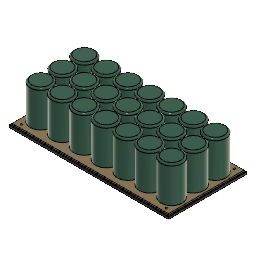
Condensadores (Autodesk Fusion 360 design; units mm, degrees)
Autodesk Fusion 360 part; units mm, degrees
sketch "Esboço1" plane through (0, 0, 0) normal (0, 0, 1) x (1, 0, 0)
  line L0 (0, 0) -> (230, 0)
  line L1 (230, 0) -> (230, 113)
  line L2 (230, 113) -> (0, 113)
  line L3 (0, 113) -> (0, 0)
  dimension "d1" = 230
  dimension "d2" = 113
  constraint horizontal L0
  constraint vertical L1
  constraint horizontal L2
  constraint vertical L3
  constraint coincident L0.start L3.end
  measures "d1" distance of L1.end L2.end
  measures "d2" distance of L0.start L2.end
extrude "Extrusão1" add sketch "Esboço1" along normal blind 3.5 makes body 1
sketch "Esboço2" plane through (0, 0, 3.5) normal (0, 0, 1) x (-1, 0, 0)
  line L0 (0, -113) -> (0, 0)
  line L1 (0, 0) -> (-230, 0)
  line L2 (-230, 0) -> (-230, -113)
  line L3 (-230, -113) -> (0, -113)
  line L4 (-2, -111) -> (-228, -111)
  line L5 (-228, -111) -> (-228, -2)
  line L6 (-228, -2) -> (-2, -2)
  line L7 (-2, -2) -> (-2, -111)
  line L8 (0, -113) -> (0, 0)
  line L9 (-230, -113) -> (0, -113)
  line L10 (-230, 0) -> (-230, -113)
  line L11 (0, 0) -> (-230, 0)
  circle A0 centre (-10.5, -105.5) radius 1.5
  circle A1 centre (-219.5, -105.5) radius 1.5
  circle A2 centre (-10.5, -7.5) radius 1.5
  circle A3 centre (-219.5, -7.5) radius 1.5
  circle A4 centre (-209.5, -88) radius 15.25
  circle A5 centre (-209.5, -56.5) radius 15.25
  circle A6 centre (-209.5, -25) radius 15.25
  line L12 (-209.5, -88) -> (-209.5, -56.5) construction
  line L13 (-209.5, -56.5) -> (-209.5, -25) construction
  line L14 (-209.5, -88) -> (-2, -88) construction
  line L15 (-209.5, -25) -> (-2, -25) construction
  line L16 (-209.5, -56.5) -> (-2, -56.5) construction
  circle A7 centre (-20.5, -88) radius 15.25
  circle A8 centre (-20.5, -56.5) radius 15.25
  circle A9 centre (-20.5, -25) radius 15.25
  circle A10 centre (-52, -25) radius 15.25
  circle A11 centre (-83.5, -25) radius 15.25
  circle A12 centre (-146.5, -25) radius 15.25
  circle A13 centre (-178, -25) radius 15.25
  circle A14 centre (-178, -56.5) radius 15.25
  circle A15 centre (-115, -56.5) radius 15.25
  circle A16 centre (-146.5, -56.5) radius 15.25
  circle A17 centre (-83.5, -56.5) radius 15.25
  circle A18 centre (-52, -56.5) radius 15.25
  circle A19 centre (-52, -88) radius 15.25
  circle A20 centre (-83.5, -88) radius 15.25
  circle A21 centre (-115, -88) radius 15.25
  circle A22 centre (-146.5, -88) radius 15.25
  circle A23 centre (-178, -88) radius 15.25
  circle A24 centre (-115, -25) radius 15.25
  line L17 (-178, -88) -> (-178, -2) construction
  line L18 (-146.5, -88) -> (-146.5, -2) construction
  line L19 (-115, -88) -> (-115, -2) construction
  line L20 (-83.5, -88) -> (-83.5, -2) construction
  line L21 (-52, -88) -> (-52, -2) construction
  line L22 (-20.5, -88) -> (-20.5, -2) construction
  dimension "d5" = 2
  dimension "d6" = 2
  dimension "d7" = 2
  dimension "d8" = 2
  dimension "d9" = 3
  dimension "d10" = 3
  dimension "d11" = 3
  dimension "d12" = 3
  dimension "d13" = 10.5
  dimension "d14" = 7.5
  dimension "d15" = 10.5
  dimension "d16" = 7.5
  dimension "d17" = 7.5
  dimension "d18" = 10.5
  dimension "d19" = 10.5
  dimension "d20" = 7.5
  dimension "d21" = 30.5
  dimension "d22" = 18.5
  dimension "d23" = 23
  dimension "d24" = 23
  dimension "d25" = 31.5
  dimension "d26" = 31.5
  dimension "d27" = 31.5
  dimension "d28" = 31.5
  dimension "d29" = 31.5
  dimension "d30" = 31.5
  dimension "d31" = 31.5
  dimension "d32" = 31.5
  constraint horizontal L4
  constraint vertical L5
  constraint horizontal L6
  constraint vertical L7
  constraint equal A4 A6
  constraint equal A4 A5
  constraint coincident A4.centre L12.start
  constraint coincident A5.centre L12.end
  constraint coincident A6.centre L13.end
  constraint vertical L12
  constraint vertical L13
  constraint coincident L7 L14.end
  constraint perpendicular L7 L14
  constraint coincident L7 L15.end
  constraint perpendicular L7 L15
  constraint coincident L7 L16.end
  constraint coincident L14 A7.centre
  constraint coincident L16 A8.centre
  constraint coincident L15 A9.centre
  constraint coincident L15 A10.centre
  constraint coincident L15 A11.centre
  constraint coincident L15 A13.centre
  constraint coincident L16 A14.centre
  constraint coincident L16 A18.centre
  constraint coincident L14 A19.centre
  constraint coincident L14 A20.centre
  constraint coincident L14 A21.centre
  constraint coincident L14 A22.centre
  constraint coincident L14 A23.centre
  constraint equal A22 A23
  constraint equal A21 A22
  constraint equal A20 A21
  constraint equal A19 A20
  constraint equal A7 A19
  constraint equal A4 A7
  constraint coincident L16 A15.centre
  constraint equal A8 A18
  constraint equal A8 A17
  constraint equal A15 A17
  constraint equal A15 A16
  constraint equal A14 A16
  constraint equal A5 A14
  constraint coincident L15 A12.centre
  constraint coincident L15 A24.centre
  constraint equal A9 A10
  constraint equal A10 A11
  constraint equal A11 A24
  constraint equal A12 A24
  constraint equal A12 A13
  constraint equal A6 A13
  constraint coincident A23.centre L17.start
  constraint coincident L6 L17.end
  constraint perpendicular L6 L17
  constraint coincident A22.centre L18.start
  constraint coincident L6 L18.end
  constraint perpendicular L6 L18
  constraint coincident A21.centre L19.start
  constraint midpoint L6 L19.end
  constraint coincident A20.centre L20.start
  constraint coincident L6 L20.end
  constraint perpendicular L6 L20
  constraint coincident A19.centre L21.start
  constraint coincident L6 L21.end
  constraint perpendicular L6 L21
  constraint coincident A7.centre L22.start
  constraint coincident L6 L22.end
  constraint perpendicular L6 L22
  constraint coincident A14.centre L17
  constraint coincident A13.centre L17
  constraint horizontal L16
  constraint coincident L16 A16.centre
  constraint coincident A16.centre L18
  constraint coincident A12.centre L18
  constraint coincident A15.centre L19
  constraint coincident A24.centre L19
  constraint coincident A17.centre L20
  constraint coincident A11.centre L20
  constraint coincident A10.centre L21
  constraint coincident A18.centre L21
  constraint coincident L16 A17.centre
  constraint coincident A9.centre L22
  constraint coincident A8.centre L22
  measures "d5" distance of L7 L8
  measures "d6" distance of L4 L9
  measures "d7" distance of L5 L10
  measures "d8" distance of L6 L11
  measures "d9" diameter of A0
  measures "d10" diameter of A1
  measures "d11" diameter of A3
  measures "d12" diameter of A2
  measures "d13" distance of L10 A1.centre
  measures "d14" distance of L9 A1.centre
  measures "d15" distance of L10 A3.centre
  measures "d16" distance of L11 A3.centre
  measures "d17" distance of L11 A2.centre
  measures "d18" distance of L8 A2.centre
  measures "d19" distance of L8 A0.centre
  measures "d20" distance of L9 A0.centre
  measures "d21" diameter of A4
  measures "d22" distance of L5 A4.centre
  measures "d23" distance of L4 A4.centre
  measures "d24" distance of L6 A6.centre
  measures "d25" distance of A4.centre A5.centre
  measures "d26" distance of A5.centre A6.centre
  measures "d27" distance of A4.centre A23.centre
  measures "d28" distance of A22.centre A23.centre
  measures "d29" distance of A21.centre A22.centre
  measures "d30" distance of A20.centre A21.centre
  measures "d31" distance of A19.centre A20.centre
  measures "d32" distance of A7.centre A19.centre
extrude "Extrusão2" add sketch "Esboço2" along normal blind 2 separate body contours L4 L5 L6 L7 makes body 2
extrude "Extrusão3" add sketch "Esboço2" along normal blind 54.1 separate body contours A4 | A5 | A6 | A7 | A8 | A9 | A10 | A11 | A12 | A13 | A14 | A15 | A16 | A17 | A18 | A19 | A20 | A21 | A22 | A23 | A24 makes body 3 at (36.8258, 58.0184, 21.5333) makes body 4 at (99.8258, 58.0184, 21.5333) makes body 5 at (131.3258, 26.5184, 21.5333) makes body 6 at (194.3258, 89.5184, 21.5333) makes body 7 at (68.3258, 89.5184, 21.5333) makes body 8 at (36.8258, 89.5184, 21.5333) makes body 9 at (162.8258, 89.5184, 21.5333) makes body 10 at (131.3258, 58.0184, 21.5333) makes body 11 at (99.8258, 26.5184, 21.5333) makes body 12 at (36.8258, 26.5184, 21.5333) makes body 13 at (5.3258, 58.0184, 21.5333) makes body 14 at (68.3258, 58.0184, 21.5333) makes body 15 at (162.8258, 26.5184, 21.5333) makes body 16 at (194.3258, 58.0184, 21.5333) makes body 17 at (99.8258, 89.5184, 21.5333) makes body 18 at (5.3258, 89.5184, 21.5333) makes body 19 at (131.3258, 89.5184, 21.5333) makes body 20 at (162.8258, 58.0184, 21.5333) makes body 21 at (194.3258, 26.5184, 21.5333) makes body 22 at (68.3258, 26.5184, 21.5333) makes body 23 at (5.3258, 26.5184, 21.5333)
extrude "Extrusão4" cut sketch "Esboço2" against normal blind 25 contours A0 | A1 | A2 | A3 bodies 1
fillet "Arredondamento1" radius 2.5 21 edges at (66.218, 62.0146, 57.6) (129.218, 62.0146, 57.6) (160.718, 30.5146, 57.6) (223.718, 93.5146, 57.6) (97.718, 93.5146, 57.6) (66.218, 93.5146, 57.6) (192.218, 93.5146, 57.6) (160.718, 62.0146, 57.6) (129.218, 30.5146, 57.6) (66.218, 30.5146, 57.6) (34.718, 62.0146, 57.6) (97.718, 62.0146, 57.6) (192.218, 30.5146, 57.6) (223.718, 62.0146, 57.6) (129.218, 93.5146, 57.6) (34.718, 93.5146, 57.6) (160.718, 93.5146, 57.6) (192.218, 62.0146, 57.6) (223.718, 30.5146, 57.6) (97.718, 30.5146, 57.6) (34.718, 30.5146, 57.6) on bodies 3 4 5 6 7 8 9 10 11 12 13 14 15 16 17 18 19 20 21 22 23
equation "d10 = d9"
equation "d11 = d9"
equation "d12 = d9"
equation "d15 = d13"
equation "d16 = d14"
equation "d17 = d14"
equation "d18 = d13"
equation "d19 = d13"
equation "d20 = d14"
equation "d24 = d23"
equation "d28 = d27"
equation "d29 = d27"
equation "d30 = d27"
equation "d31 = d27"
equation "d32 = d27"
equation "d35 = 52.1 mm + 2 mm"
